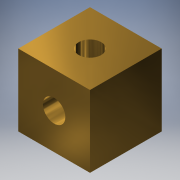
# Autodesk Inventor part: 垂直ブロック8
Saved by Autodesk Inventor 2017 (Build 210142000, 142)
## iProperties
Part Number: 垂直ブロック8
Material: 真鍮
Document SubType Name: Modeling
Designer: 雪村
Density: 8.49 g/cm^3
Appearance: 真鍮 - つや出し
Mass: 3.76851 g
Surface Area: 4.65029 cm^2
Volume: 0.443877 cm^3
Author: 雪村
Autodesk Inventor part; units mm, degrees
ref_plane "YZ Plane" through (0, 0, 0) normal (1, 0, 0) x (0, 1, 0)
ref_plane "XZ Plane" through (0, 0, 0) normal (0, 1, 0) x (-1, 0, 0)
ref_plane "XY Plane" through (0, 0, 0) normal (0, 0, 1) x (1, 0, 0)
sketch "スケッチ1" plane through (0, 0, 0) normal (0, 0, 1) x (1, 0, 0)
  line L0 (4, 4) -> (4, -4)
  line L1 (4, -4) -> (-4, -4)
  line L2 (-4, -4) -> (-4, 4)
  line L3 (-4, 4) -> (4, 4)
  circle A0 centre (0, 0) radius 1.25
  dimension "d0" = 8
  dimension "d1" = 2.5
  constraints: 8 end point, 2 coincident, 1 centre point, 1 horizontal, 9 other
  measures "d0" distance of L0.end L1.end
  measures "d1" diameter of A0
extrude "押し出し1" add sketch "スケッチ1" along normal blind 8
sketch "スケッチ2" plane through (-4, 4, 0) normal (0, 1, 0) x (1, 0, 0)
  line L0 (0, 0) -> (8, 0) projected
  line L1 (0, 0) -> (0, -8) projected
  line L2 (8, -8) -> (0, -8) projected
  line L3 (8, 0) -> (8, -8) projected
  circle A0 centre (4, -4) radius 4
  circle A1 centre (4, -4) radius 1.25
  line L4 (0, 0) -> (8, 0) projected
  line L5 (8, 0) -> (8, -8) projected
  point P0 (4, 0)
  dimension "d4" = 8
  dimension "d5" = 2.5
  constraints: 2 centre point, 2 tangent, 1 coincident
  measures "d4" diameter of A0
  measures "d5" diameter of A1
extrude "押し出し2" cut sketch "スケッチ2" against normal blind 8 contours A1
